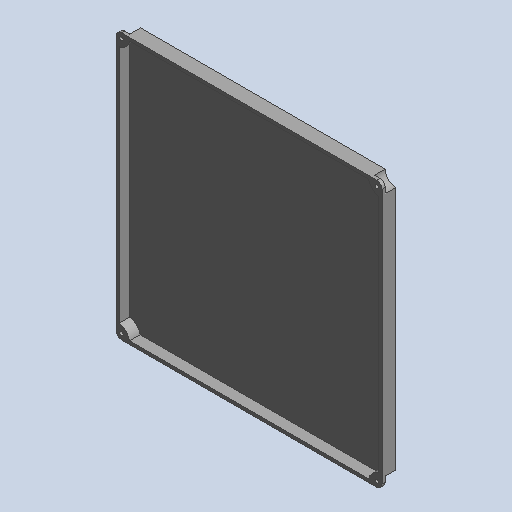
# Autodesk Inventor part: Enclosure cover
Saved by Autodesk Inventor 2026 (Build 300175050, 175E)
## iProperties
Part Number: Enclosure cover
Material: Generic
Document SubType Name: Modeling
Designer: Kartik
Mass: 216.415 g
Surface Area: 1473.79 cm^2
Volume: 216.415 cm^3
Density: 1 g/cm^3
Appearance: Default
Author: Kartik
Autodesk Inventor part; units mm, degrees
ref_plane "YZ Plane" through (0, 0, 0) normal (1, 0, 0) x (0, 1, 0)
ref_plane "XZ Plane" through (0, 0, 0) normal (0, 1, 0) x (-1, 0, 0)
ref_plane "XY Plane" through (0, 0, 0) normal (0, 0, 1) x (1, 0, 0)
sketch "Sketch1" plane through (0, 0, 0) normal (0, 0, 1) x (1, 0, 0)
  line L0 (-123.0769, 96.9231) -> (116.9231, 96.9231)
  line L1 (116.9231, 86.9231) -> (116.9231, -153.0769)
  line L2 (106.9231, -153.0769) -> (-123.0769, -153.0769)
  line L3 (-133.0769, -143.0769) -> (-133.0769, 96.9231)
  arc A0 (-133.0769, 86.9231) -> (-123.0769, 96.9231) centre (-133.0769, 96.9231) ccw
  arc A1 (106.9231, 96.9231) -> (116.9231, 86.9231) centre (116.9231, 96.9231) ccw
  arc A2 (116.9231, -143.0769) -> (106.9231, -153.0769) centre (116.9231, -153.0769) ccw
  arc A3 (-123.0769, -153.0769) -> (-133.0769, -143.0769) centre (-133.0769, -153.0769) ccw
  point P0 (0, 0)
  dimension "d0" = 250
  dimension "d1" = 250
  dimension "d4" = 20
  dimension "d5" = 20
  dimension "d6" = 20
  dimension "d7" = 20
  constraints: 8 end point, 8 point on circle, 4 centre point, 3 coincident, 3 point on line, 2 parallel, 1 horizontal, 1 perpendicular
  measures "d0" distance of L3.end L0.end
  measures "d1" distance of L0.end L1.end
  measures "d4" diameter of A0
  measures "d5" diameter of A1
  measures "d6" diameter of A2
  measures "d7" diameter of A3
extrude "Extrusion1" add sketch "Sketch1" along normal blind 3
sketch "Sketch2" plane through (0, 0, 3) normal (0, 0, 1) x (1, 0, 0)
  line L0 (-123.0769, -153.0769) -> (106.9231, -153.0769) projected
  arc A0 (116.9231, -143.0769) -> (106.9231, -153.0769) centre (116.9231, -153.0769) ccw projected
  line L1 (116.9231, -143.0769) -> (116.9231, 86.9231) projected
  arc A1 (106.9231, 96.9231) -> (116.9231, 86.9231) centre (116.9231, 96.9231) ccw projected
  line L2 (106.9231, 96.9231) -> (-123.0769, 96.9231) projected
  arc A2 (-133.0769, 86.9231) -> (-123.0769, 96.9231) centre (-133.0769, 96.9231) ccw projected
  line L3 (-133.0769, 86.9231) -> (-133.0769, -143.0769) projected
  arc A3 (-123.0769, -153.0769) -> (-133.0769, -143.0769) centre (-133.0769, -153.0769) ccw projected
  line L4 (-120.4278, 93.9231) -> (104.274, 93.9231)
  arc A4 (104.274, 93.9231) -> (113.9231, 84.274) centre (116.9231, 96.9231) ccw
  line L5 (113.9231, 84.274) -> (113.9231, -140.4278)
  arc A5 (113.9231, -140.4278) -> (104.274, -150.0769) centre (116.9231, -153.0769) ccw
  line L6 (104.274, -150.0769) -> (-120.4278, -150.0769)
  arc A6 (-120.4278, -150.0769) -> (-130.0769, -140.4278) centre (-133.0769, -153.0769) ccw
  line L7 (-130.0769, -140.4278) -> (-130.0769, 84.274)
  arc A7 (-130.0769, 84.274) -> (-120.4278, 93.9231) centre (-133.0769, 96.9231) ccw
  point P0 (0, 0)
  dimension "d8" = 3
  constraints: 8 end point, 8 point on circle, 4 centre point, 7 other
  measures "d8" distance between parallel lines of L2 L4
extrude "Extrusion2" add sketch "Sketch2" along normal blind 10
sketch "Sketch3" plane through (0, 0, 13) normal (0, 0, 1) x (1, 0, 0)
  line L0 (106.9231, 96.9231) -> (-123.0769, 96.9231) projected
  line L1 (-133.0769, 86.9231) -> (-133.0769, -143.0769) projected
  line L2 (116.9231, -143.0769) -> (116.9231, 86.9231) projected
  line L3 (-123.0769, -153.0769) -> (106.9231, -153.0769) projected
  arc A0 (116.9231, -143.0769) -> (106.9231, -153.0769) centre (116.9231, -153.0769) ccw projected
  arc A1 (-123.0769, -153.0769) -> (-133.0769, -143.0769) centre (-133.0769, -153.0769) ccw projected
  arc A2 (-133.0769, 86.9231) -> (-123.0769, 96.9231) centre (-133.0769, 96.9231) ccw projected
  arc A3 (106.9231, 96.9231) -> (116.9231, 86.9231) centre (116.9231, 96.9231) ccw projected
  line L4 (-133.0769, 96.9231) -> (116.9231, 96.9231)
  line L5 (116.9231, 96.9231) -> (116.9231, -153.0769)
  line L6 (116.9231, -153.0769) -> (-133.0769, -153.0769)
  line L7 (-133.0769, -153.0769) -> (-133.0769, 96.9231)
  point P0 (0, 0)
  point P1 (106.9231, -153.0769)
  constraints: 8 end point, 2 parallel, 1 horizontal, 1 perpendicular
extrude "Extrusion3" add sketch "Sketch3" against normal blind 3 contours L4 L5 A3 | A2 L7 L4 | L5 L6 A0 | A1 L6 L7
fillet "Fillet1" radius 5 4 edges at (116.9231, -153.0769, 11.5) (-133.0769, -153.0769, 11.5) (116.9231, 96.9231, 11.5) (-133.0769, 96.9231, 11.5)
sketch "Sketch4" plane through (0, 0, 13) normal (0, 0, 1) x (1, 0, 0)
  arc A0 (-128.0769, 96.9231) -> (-133.0769, 91.9231) centre (-128.0769, 91.9231) ccw projected
  line L0 (-133.0769, 91.9231) -> (-133.0769, -148.0769) projected
  arc A1 (-133.0769, -148.0769) -> (-128.0769, -153.0769) centre (-128.0769, -148.0769) ccw projected
  line L1 (-128.0769, -153.0769) -> (111.9231, -153.0769) projected
  arc A2 (111.9231, -153.0769) -> (116.9231, -148.0769) centre (111.9231, -148.0769) ccw projected
  line L2 (116.9231, -148.0769) -> (116.9231, 91.9231) projected
  arc A3 (116.9231, 91.9231) -> (111.9231, 96.9231) centre (111.9231, 91.9231) ccw projected
  line L3 (111.9231, 96.9231) -> (-128.0769, 96.9231) projected
  line L4 (-120.4278, 93.9231) -> (104.274, 93.9231) projected
  arc A4 (104.274, 93.9231) -> (113.9231, 84.274) centre (116.9231, 96.9231) ccw projected
  line L5 (113.9231, 84.274) -> (113.9231, -140.4278) projected
  arc A5 (113.9231, -140.4278) -> (104.274, -150.0769) centre (116.9231, -153.0769) ccw projected
  line L6 (104.274, -150.0769) -> (-120.4278, -150.0769) projected
  arc A6 (-120.4278, -150.0769) -> (-130.0769, -140.4278) centre (-133.0769, -153.0769) ccw projected
  line L7 (-130.0769, -140.4278) -> (-130.0769, 84.274) projected
  arc A7 (-130.0769, 84.274) -> (-120.4278, 93.9231) centre (-133.0769, 96.9231) ccw projected
  circle A8 centre (-128.0769, 91.9231) radius 1.6
  circle A9 centre (-128.0769, -148.0769) radius 1.6
  circle A10 centre (111.9231, 91.9231) radius 1.6
  circle A11 centre (111.9231, -148.0769) radius 1.6
  point P0 (0, 0)
  dimension "d14" = 3.2
  dimension "d15" = 5
  dimension "d16" = 5
  dimension "d19" = 240
  dimension "d22" = 240
  constraints: 4 centre point, 1 horizontal, 1 vertical, 6 other
  measures "d14" diameter of A8
  measures "d15" distance from line of L3 A8.centre
  measures "d16" distance from line of A8.centre L0
  measures "d19" distance of A8.centre A9.centre
  measures "d22" distance of A8.centre A10.centre
extrude "Extrusion4" cut sketch "Sketch4" against normal blind 3 contours A8 | A9 | A10 | A11
body "Solid1"
